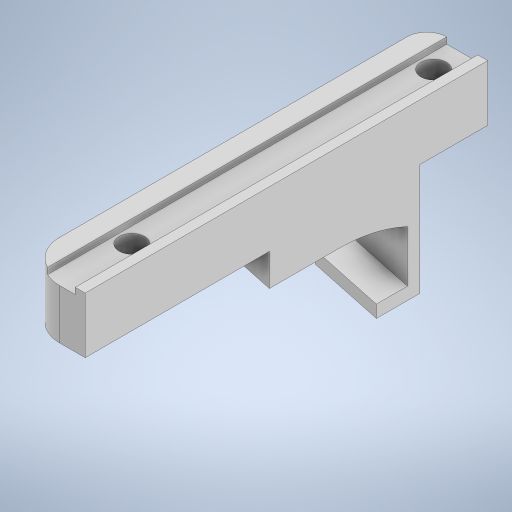
# Autodesk Inventor part: Right-Brush-Top
Saved by Autodesk Inventor 2024 (Build 280153000, 153)
## iProperties
Created: 2023-12-13
Part Number: Right-Brush-Top
Material: Generic
Document SubType Name: Modeling
Designer: shaun
Density: 1 g/cm^3
Appearance: Default
Author: shaun
Autodesk Inventor part; units mm, degrees
ref_plane "YZ Plane" through (0, 0, 0) normal (1, 0, 0) x (0, 1, 0)
sketch "Sketch1" plane through (0, 0, 0) normal (0, 1, 0) x (-1, 0, 0)
  line L0 (0, 64.7) -> (11.4, 64.7) construction
  line L1 (11.4, 64.7) -> (11.4, 0) construction
  line L2 (11.4, 0) -> (0, 0) construction
  line L3 (0, 0) -> (0, 64.7) construction
  line L4 (5.7, 64.7) -> (5.7, 0) construction
  line L5 (11.4, 32.35) -> (0, 32.35) construction
  circle A0 centre (5.7, 53.1) radius 1.6 construction
  circle A1 centre (5.7, 53.1) radius 2.05
  circle A2 centre (5.7, 43.4) radius 1.6 construction
  circle A3 centre (5.7, 43.4) radius 2.05 construction
  circle A4 centre (5.7, 33.7) radius 1.6 construction
  circle A5 centre (5.7, 33.7) radius 2.05 construction
  circle A6 centre (5.7, 24) radius 1.6 construction
  circle A7 centre (5.7, 24) radius 2.05 construction
  circle A8 centre (5.7, 14.3) radius 1.6 construction
  circle A9 centre (5.7, 14.3) radius 2.05 construction
  circle A10 centre (5.7, 4.6) radius 1.6 construction
  circle A11 centre (5.7, 4.6) radius 2.05
  line L6 (8.2, 64.7) -> (3.2, 64.7) construction
  line L7 (3.2, 64.7) -> (3.2, 0)
  line L8 (3.2, 0) -> (8.2, 0) construction
  line L9 (8.2, 0) -> (8.2, 64.7)
  circle A12 centre (5.7, 53.1) radius 2.5 construction
  circle A13 centre (5.7, 59) radius 5.7 construction
  circle A14 centre (8.2, 3.2) radius 3.2 construction
  line L10 (0, 0) -> (3.2, 0) construction
  line L11 (1.6, 0) -> (1.6, 64.7)
  circle A15 centre (5.7, 4.6) radius 3.65
  circle A16 centre (5.7, 14.3) radius 3.65 construction
  circle A17 centre (5.7, 24) radius 3.65 construction
  circle A18 centre (5.7, 33.7) radius 3.65 construction
  circle A19 centre (5.7, 43.4) radius 3.65 construction
  circle A20 centre (5.7, 53.1) radius 3.65
  arc A21 (8.2, 0) -> (11.4, 3.2) centre (8.2, 3.2) ccw
  arc A22 (11.4, 59) -> (5.7, 64.7) centre (5.7, 59) ccw
  line L12 (11.4, 3.2) -> (11.4, 59)
  line L13 (1.6, 0) -> (8.2, 0)
  line L14 (1.6, 64.7) -> (5.7, 64.7)
  point P0 (5.7, 54.7)
  point P1 (5.7, 3)
  point P2 (-5.6396, 32.0975)
  point P3 (-5.6396, -32.6025)
  point P4 (-1.0396, 31.5935)
  point P5 (8.2, 64.1225)
  point P6 (8.2, 55.7594)
  point P7 (8.2, 50.4406)
  point P8 (3.2, 0)
  point P9 (3.2, 50.4406)
  point P10 (3.2, 55.7594)
  dimension "d4" = 3.2
  dimension "d5" = 4.1
  dimension "d6" = 9.7
  dimension "d7" = 6.5
  dimension "d8" = 10
  dimension "d9" = 3
  dimension "d10" = 0.9
  dimension "d11" = 3.2
  dimension "d12" = 7.3
  constraints: 30 end point, 21 centre point, 17 coincident, 10 point on line, 8 point on circle, 5 equal radius, 5 midpoint, 5 parallel, 5 tangent, 3 perpendicular, 2 collinear, 2 horizontal, 2 line through centre, 2 vertical, 2 vertical alignment, 22 other
  measures "d5" diameter of A1
  measures "d6" distance of point (5.7, 53.1) A2.centre
  measures "d8" distance from line of L0 point (5.7, 54.7)
  measures "d9" distance of L4.end point (5.7, 3)
  measures "d11" distance between parallel lines of L1 L9
  measures "d12" diameter of A15
extrude "Extrusion1" add sketch "Sketch1" along normal blind 6 contours L7 A20 A15 L13 L11 L14 | L7 A20 | A20 L9 | L9 A22 L12 A21 A15 A20 | L7 A15 | A15 L9
extrude "Extrusion2" add sketch "Sketch1" along normal blind 5 contours L14 A22 L9 A20 L7 | A20 L9 L7 | A20 L9 A15 L7 | A15 L9 L7 | L7 A15 L9 L13
extrude "Extrusion3" add sketch "Sketch1" against normal blind 3 contours L14 A22 L9 A20 L7 | L7 A20 A15 L13 L11 L14 | A20 L9 A15 L7 | L9 A22 L12 A21 A15 A20 | L7 A15 L9 L13
sketch "Sketch2" plane through (0, -3, 0) normal (0, -1, 0) x (1, 0, 0)
  line L0 (-5.7, 53.1) -> (-5.7, 4.6) construction
  circle A0 centre (-5.7, 53.1) radius 4.85 construction
  circle A1 centre (-5.7, 43.4) radius 4.85 construction
  circle A2 centre (-5.7, 33.7) radius 4.85 construction
  circle A3 centre (-5.7, 24) radius 4.85 construction
  circle A4 centre (-5.7, 14.3) radius 4.85 construction
  circle A5 centre (-5.7, 4.6) radius 4.85 construction
  line L1 (-11.4, 3.2) -> (-11.4, 59) construction
  line L2 (0, 35.1) -> (-11.4, 35.1) construction
  line L3 (-11.4, 35.1) -> (-11.4, 12.9) construction
  line L4 (-11.4, 12.9) -> (0, 12.9) construction
  line L5 (0, 12.9) -> (0, 35.1) construction
  line L6 (0, 35.1) -> (-11.4, 12.9) construction
  line L7 (-11.4, 35.1) -> (0, 12.9) construction
  point P0 (0, 0)
  dimension "d20" = 22.2
  constraints: 14 end point, 10 equal radius, 7 coincident, 6 centre point, 5 point on line, 2 midpoint, 2 parallel, 1 horizontal, 1 perpendicular, 1 vertical
  measures "d20" distance between parallel lines of L4 L2
ref_plane "Work Plane1" through (-11.4, -3, 12.9) normal (0, 0, -1) x (-1, 0, 0)
sketch "Sketch3" plane through (-11.4, -3, 12.9) normal (0, 0, -1) x (-1, 0, 0)
  line L0 (0, 0) -> (-9.8, 0)
  line L1 (0, 0) -> (9.8, 0) construction
  line L2 (9.8, 0) -> (9.8, -2.4) construction
  line L3 (0, 0) -> (0, -15.3081)
  line L4 (0, -15.3081) -> (-9.8, -17.934)
  line L5 (-9.8, -17.934) -> (-9.8, 0)
  line L6 (-9.8, -15.934) -> (0, -13.3081)
  line L7 (9.8, -2.4) -> (0, -5.0259) construction
  line L8 (0, -5.0259) -> (-9.8, -7.6518)
  line L9 (9.8, -2.4) -> (0, -2.4) construction
  line L10 (0, -13.3081) -> (-2.0706, -5.5807) construction
  point P0 (-11.4, 3)
  dimension "d32" = 2.4
  dimension "d34" = 15
  dimension "d35" = 8
  dimension "d36" = 2
  constraints: 22 end point, 6 point on line, 3 parallel, 3 perpendicular, 2 collinear, 2 horizontal, 1 vertical
  measures "d32" distance of L2.end L1.end
  measures "d34" angle of L9 L7
  measures "d35" distance of L6.end L10.end
  measures "d36" distance of L3.end L6.end
extrude "Extrusion4" add sketch "Sketch3" along normal blind 2
extrude "Extrusion5" add sketch "Sketch3" against normal blind 22.2 contours L3 L8 L5 L0
extrude "Extrusion6" add sketch "Sketch3" against normal blind 5 contours L3 L4 L5 L6
ref_plane "Work Plane3" through (-9.3294, -8.5807, 12.9) normal (-0.9659258, 0.258819, 0) x (-0.258819, -0.9659258, 0)
sketch "Sketch5" plane through (-9.3294, -8.5807, 12.9) normal (-0.9659258, 0.258819, 0) x (-0.258819, -0.9659258, 0)
  line L0 (0, 0) -> (0, 22.2) projected
  arc A0 (0, 22.2) -> (0, 0) centre (24.4688, 11.1) ccw
  line L1 (-2.4, 11.1) -> (-2.4, 22.2)
  line L2 (-2.4, 22.2) -> (0, 22.2)
  line L3 (-4.8546, 22.2) -> (0, 22.2) projected
  point P0 (-10.703, -12.9)
  point P1 (0, 11.1)
  dimension "d37" = 2.4
  constraints: 4 end point, 3 point on circle, 1 centre point, 1 midpoint, 1 point on line, 1 vertical
  measures "d37" distance of L1.start point (0, 11.1)
extrude "Extrusion7" cut sketch "Sketch5" along normal through all both and the other way through all
body "Solid1"
